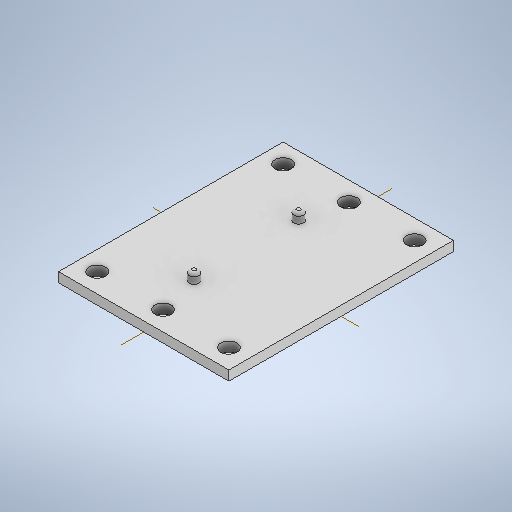
# Autodesk Inventor part: connector-houseing-bottom-plate
Saved by Autodesk Inventor 2025 (Build 290162000, 162)
## iProperties
Created: 2025-05-30
Part Number: connector-houseing-bottom-plate
Material: Generic
Document SubType Name: Modeling
Designer: mumin
Density: 1 g/cm^3
Appearance: Default
Author: mumin
Autodesk Inventor part; units mm, degrees
ref_plane "YZ Plane" through (0, 0, 0) normal (1, 0, 0) x (0, 1, 0)
ref_plane "XZ Plane" through (0, 0, 0) normal (0, 1, 0) x (-1, 0, 0)
ref_plane "XY Plane" through (0, 0, 0) normal (0, 0, 1) x (1, 0, 0)
sketch "Sketch1" plane through (0, 0, 0) normal (0, 1, 0) x (-1, 0, 0)
  line L0 (22, 29) -> (-22, 29)
  line L1 (-22, 29) -> (-22, -29)
  line L2 (-22, -29) -> (22, -29)
  line L3 (22, -29) -> (22, 29)
  point P0 (0, 0)
  point P1 (0, -29)
  dimension "d2" = 44
  dimension "d3" = 58
  constraints: 8 end point, 2 parallel, 1 horizontal, 1 midpoint, 1 perpendicular
  measures "d2" distance of L2.end L1.end
  measures "d3" distance of L1.end L0.end
extrude "Extrusion1" add sketch "Sketch1" along normal blind 2.5
sketch "Sketch2" plane through (0, 2.5, 0) normal (0, 1, 0) x (1, 0, 0)
  line L0 (0, 40.6) -> (0, -40.6) projected
  line L1 (22, 29) -> (-22, 29) projected
  point P0 (0, 0)
  point P1 (0, 24)
  dimension "d22" = 5
  constraints: 1 point on line
  measures "d22" distance from line of L1 point (0, 24)
hole "Hole1" at (0, 2.5, -24) direction (0, -1, 0) diameter 4.2 end through all
pattern_linear "Rectangular Pattern1" count 2 spacing 17 along (-1, 0, 0) count 2 spacing 17 along (1, 0, 0) of "Hole1"
mirror "Mirror1" about plane through (0, 0, 0) normal (0, 0, 1) of "Hole1", "Rectangular Pattern1"
sketch "Sketch3" plane through (0, 2.5, 0) normal (0, 1, 0) x (1, 0, 0)
  circle A0 centre (-2.5, 13.5) radius 1.25
  line L0 (0, 40.6) -> (0, -40.6) projected
  line L1 (-30.8, 0) -> (30.8, 0) projected
  circle A1 centre (-2.5, -13.5) radius 1.25
  point P0 (0, 0)
  dimension "d29" = 2.5
  dimension "d30" = 2.5
  dimension "d31" = 13.5
  constraints: 2 centre point, 1 symmetric about line, 1 other
  measures "d29" diameter of A0
  measures "d30" distance from line of L0 A0.centre
  measures "d31" distance from line of L1 A0.centre
extrude "Extrusion2" add sketch "Sketch3" along normal blind 2.5
fillet "Fillet1" radius 0.75 2 edges at (-3.75, 5, -13.5) (-3.75, 5, 13.5)
body "Solid1"
